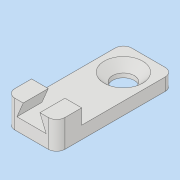
# Autodesk Inventor part: HallEffectSpoolSensorMount
Saved by Autodesk Inventor 2017 (Build 210142000, 142)
## iProperties
Created: 2018-04-12
Part Number: HallEffectSpoolSensorMount
Material: ABS Plastic
Document SubType Name: Modeling
Designer: Derek Wider
Density: 1.06 g/cm^3
Appearance: Smooth - White
Author: Derek Wider
Autodesk Inventor part; units mm, degrees
ref_plane "YZ Plane" through (0, 0, 0) normal (1, 0, 0) x (0, 1, 0)
ref_plane "XZ Plane" through (0, 0, 0) normal (0, 1, 0) x (-1, 0, 0)
ref_plane "XY Plane" through (0, 0, 0) normal (0, 0, 1) x (1, 0, 0)
sketch "Sketch1" plane through (0, 0, 0) normal (0, 1, 0) x (-1, 0, 0)
  line L0 (0, 0) -> (7.62, 0)
  line L1 (7.62, 0) -> (7.62, -17.78)
  line L2 (7.62, -17.78) -> (0, -17.78)
  line L3 (0, -17.78) -> (0, 0)
  dimension "d0" = 7.62
  dimension "d1" = 17.78
  constraints: 8 end point, 2 parallel, 1 horizontal, 1 perpendicular
  measures "d0" distance of L0.start L0.end
  measures "d1" distance of L0.end L1.end
extrude "Extrusion1" add sketch "Sketch1" along normal blind 1.905
sketch "Sketch3" plane through (-7.62, 0, 0) normal (0, 0, 1) x (1, 0, 0)
  line L0 (0, 1.905) -> (7.62, 1.905) projected
  line L1 (1.5875, 1.905) -> (2.54, 4.191)
  line L2 (2.54, 4.191) -> (0, 4.191)
  line L3 (0, 4.191) -> (0, 1.905)
  line L4 (5.08, 4.191) -> (6.0325, 1.905)
  line L5 (5.08, 4.191) -> (7.62, 4.191)
  line L6 (7.62, 4.191) -> (7.62, 1.905)
  point P0 (7.62, 0)
  dimension "d4" = 2.54
  dimension "d5" = 4.445
  dimension "d6" = 2.286
  constraints: 12 end point, 4 point on line, 2 equal length, 2 perpendicular, 1 horizontal
  measures "d4" distance of L4.start L1.end
  measures "d5" distance of L4.end L1.start
  measures "d6" distance of L2.end L0.start
extrude "Extrusion2" add sketch "Sketch3" against normal blind 3.81
sketch "Sketch4" plane through (0, 1.905, 0) normal (0, 1, 0) x (1, 0, 0)
  line L0 (0, 17.78) -> (-7.62, 17.78) projected
  circle A0 centre (-3.81, 13.97) radius 1.651
  point P0 (0, 0)
  point P1 (-3.81, 17.78)
  dimension "d9" = 3.302
  dimension "d10" = 3.81
  constraints: 1 centre point, 1 midpoint, 1 vertical alignment
  measures "d9" diameter of A0
  measures "d10" distance of point (-3.81, 17.78) A0.centre
extrude "Extrusion3" cut sketch "Sketch4" against normal through all
chamfer "Chamfer1" distance 1.27 angle 45 1 edges at (-5.461, 1.905, -13.97)
fillet "Fillet1" radius 1.27 4 edges at (0, 0.9525, -17.78) (-7.62, 0.9525, -17.78) (0, 2.0955, 0) (-7.62, 2.0955, 0)
body "Solid1"
